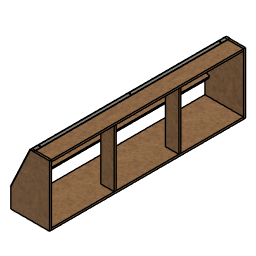
tricoro_panel (Autodesk Fusion 360 design; units mm, degrees)
Autodesk Fusion 360 part; units mm, degrees
note: some values were not read from the file. Set by a fixed rule: which sketch regions a step uses.
sketch "Sketch1" plane through (0, 0, 0) normal (0, 1, 0) x (1, 0, 0)
  line L0 (0, 0) -> (18, 0)
  line L1 (0, 0) -> (-101.4284, 217.5139)
  line L2 (0, 0) -> (240, 0) construction
  line L3 (-1.2741, -2) -> (-103.241, 216.6686)
  line L4 (-1.2741, -2) -> (18, -2)
  line L5 (18, -2) -> (18, 0)
  line L6 (-103.241, 216.6686) -> (-101.4284, 217.5139)
  dimension "d1" = 18
  dimension "d2" = 115
  dimension "d3" = 240
  dimension "d4" = -2
  constraint coincident L0.start L1.start
  constraint horizontal L0
  constraint horizontal L2
  constraint perpendicular L2 L5
  constraint perpendicular L1 L6
  measures "d1" distance of L0.start L0.end
  measures "d2" angle of L1 L2
  measures "d3" distance of L0.start L1.end
extrude "Extrude1" add sketch "Sketch1" along normal blind 1020 makes body 1
sketch "Sketch2" plane through (0, 0, 0) normal (0, -1, 0) x (1, 0, 0)
  line L0 (18, 2) -> (-1.2741, 2)
  line L1 (-1.2741, 2) -> (-103.241, -216.6686)
  line L2 (-103.241, -216.6686) -> (-101.4284, -217.5139)
  line L3 (-101.4284, -217.5139) -> (0, 0)
  line L4 (0, 0) -> (18, 0)
  line L5 (18, 0) -> (18, 2)
  line L6 (0, 0) -> (100, 0)
  line L7 (100, 0) -> (100, -220)
  line L8 (100, -220) -> (0, -220)
  line L9 (0, -220) -> (0, 0)
  line L10 (0, 0) -> (-101.4284, 0)
  line L11 (-101.4284, 0) -> (-101.4284, -217.5139)
  line L12 (-101.4284, -217.5139) -> (0, -217.5139)
  line L13 (0, -217.5139) -> (0, 0)
  line L14 (-101.4284, -217.5139) -> (100, -217.5139)
  line L15 (100, -217.5139) -> (100, -317.5139)
  line L16 (100, -317.5139) -> (-101.4284, -317.5139)
  line L17 (-101.4284, -317.5139) -> (-101.4284, -217.5139)
  dimension "d7" = 100
  dimension "d8" = 100
  constraint horizontal L6
  constraint vertical L7
  constraint horizontal L8
  constraint vertical L9
  constraint coincident L3.end L4.start
  constraint horizontal L10
  constraint vertical L11
  constraint horizontal L12
  constraint vertical L13
  constraint coincident L2.end L3.start
  constraint horizontal L14
  constraint vertical L15
  constraint horizontal L16
  constraint vertical L17
  measures "d7" distance of L3.end L6.end
  measures "d8" distance of L2.end L16.end
extrude "Extrude2" add sketch "Sketch2" against normal blind 10 separate body contours L4 L6 L7 L9 L13 L14 | L3 L9 L12 L13 L14 | L8 L9 L12 L14 L15 L16 L17 | L7 L8 L9 L14 L15 makes body 2
copy_body "CopyPasteBodies1" bodies 2 makes body 3
move_body "Move1" bodies 3 to x (1, 0, 0) y (0, 1, 0) z (0, 0, 1) at (0, 1010, 0)
sketch "Sketch3" plane through (0, 1010, 0) normal (0, -1, 0) x (1, 0, 0)
  line L0 (-101.4284, -317.5139) -> (100, -317.5139)
  line L1 (100, -317.5139) -> (100, 0)
  line L2 (100, 0) -> (0, 0)
  line L3 (0, 0) -> (-101.4284, -217.5139)
  line L4 (-101.4284, -217.5139) -> (-101.4284, -317.5139)
  line L5 (-101.4284, -217.5139) -> (-83.3022, -225.9662)
  line L6 (-83.3022, -225.9662) -> (-76.963, -212.3716)
  line L7 (-76.963, -212.3716) -> (-95.0891, -203.9193)
  line L8 (-95.0891, -203.9193) -> (-101.4284, -217.5139)
  dimension "d11" = 20
  dimension "d12" = 15
  constraint coincident L3.end L4.start
  constraint perpendicular L3 L5
  constraint perpendicular L5 L6
  constraint coincident L3 L7.end
  constraint perpendicular L3 L7
  measures "d11" distance of L3.end L5.end
  measures "d12" distance of L5.end L6.end
extrude "Extrude3" add sketch "Sketch3" along normal blind 1000 separate body contours L3 L5 L6 L7 L8 makes body 4
sketch "Sketch4" plane through (0, 1010, 0) normal (0, -1, 0) x (1, 0, 0)
  line L0 (-101.4284, -317.5139) -> (100, -317.5139)
  line L1 (100, -317.5139) -> (100, 0)
  line L2 (100, 0) -> (0, 0)
  line L3 (0, 0) -> (-101.4284, -217.5139)
  line L4 (-101.4284, -217.5139) -> (-101.4284, -317.5139)
  line L5 (100, 0) -> (0, 0)
  line L6 (0, 0) -> (0, -10)
  line L7 (0, -10) -> (100, -10)
  line L8 (100, -10) -> (100, 0)
  constraint horizontal L5
  constraint vertical L6
  constraint horizontal L7
  constraint vertical L8
  constraint coincident L1.end L2.start
extrude "Extrude4" add sketch "Sketch4" along normal blind 1000 separate body contours L1 L2 L5 L6 L7 L8 makes body 5
sketch "Sketch5" plane through (0, 1010, 0) normal (0, -1, 0) x (1, 0, 0)
  line L0 (-101.4284, -317.5139) -> (100, -317.5139)
  line L1 (100, -317.5139) -> (100, 0)
  line L2 (100, 0) -> (0, 0)
  line L3 (0, 0) -> (-101.4284, -217.5139)
  line L4 (-101.4284, -217.5139) -> (-101.4284, -317.5139)
  line L5 (100, -317.5139) -> (-101.4284, -317.5139)
  line L6 (-101.4284, -317.5139) -> (-101.4284, -307.5139)
  line L7 (-101.4284, -307.5139) -> (100, -307.5139)
  line L8 (100, -307.5139) -> (100, -317.5139)
  dimension "d17" = 10
  constraint horizontal L5
  constraint vertical L6
  constraint horizontal L7
  constraint vertical L8
  constraint coincident L0.end L1.start
  measures "d17" distance of L0.end L7.end
extrude "Extrude5" add sketch "Sketch5" along normal blind 1000 separate body contours L0 L1 L4 L5 L6 L7 L8 makes body 6
sketch "Sketch6" plane through (100, 0, 0) normal (1, 0, 0) x (0, 1, 0)
  line L0 (0, 0) -> (0, -317.5139)
  line L1 (0, -317.5139) -> (10, -317.5139)
  line L2 (10, -317.5139) -> (10, 0)
  line L3 (10, 0) -> (0, 0)
  line L4 (10, -10) -> (0, -10)
  line L5 (0, -10) -> (0, -307.5)
  line L6 (0, -307.5) -> (10, -307.5)
  line L7 (10, -307.5) -> (10, -10)
  line L8 (336.6667, -307.5) -> (346.6667, -307.5)
  line L9 (346.6667, -307.5) -> (346.6667, -10)
  line L10 (336.6667, -10) -> (336.6667, -307.5)
  line L11 (346.6667, -10) -> (336.6667, -10)
  line L12 (346.6667, 0) -> (336.6667, 0)
  line L13 (673.3333, -307.5) -> (683.3333, -307.5)
  line L14 (683.3333, -307.5) -> (683.3333, -10)
  line L15 (673.3333, -10) -> (673.3333, -307.5)
  line L16 (683.3333, -10) -> (673.3333, -10)
  line L17 (683.3333, 0) -> (673.3333, 0)
  line L18 (1010, -307.5) -> (1020, -307.5)
  line L19 (1020, -307.5) -> (1020, -10)
  line L20 (1010, -10) -> (1010, -307.5)
  line L21 (1020, -10) -> (1010, -10)
  line L22 (1020, 0) -> (1010, 0)
  point P0 (336.6667, 0)
  point P1 (673.3333, 0)
  point P2 (1010, 0)
  dimension "d22" = 1010
  dimension "d23" = 0
  constraint horizontal L4
  constraint vertical L5
  constraint horizontal L6
  constraint vertical L7
  constraint coincident L0 L5.end
  constraint coincident L2 L4.start
extrude "Extrude6" add sketch "Sketch6" against normal blind 70 separate body contours L8 L9 L10 L11 | L13 L14 L15 L16 makes body 7 at (76.6667, 336.6667, -109.1667) makes body 8 at (76.6667, 673.3333, -109.1667)
sketch "Sketch7" plane through (0, 0, 2) normal (0, 0, 1) x (-1, 0, 0)
  line L0 (1.2741, 0) -> (-18, 0)
  line L1 (-18, 0) -> (-18, -1020)
  line L2 (-18, -1020) -> (1.2741, -1020)
  line L3 (1.2741, -1020) -> (1.2741, 0)
  line L4 (-18, 0) -> (-8, 0)
  line L5 (-8, 0) -> (-8, -40)
  line L6 (-8, -40) -> (-18, -40)
  line L7 (-18, -40) -> (-18, 0)
  circle A0 centre (-8, -40) radius 3
  circle A1 centre (-8, -510) radius 3
  circle A2 centre (-8, -980) radius 3
  point P0 (-8, -510)
  point P1 (-8, -980)
  dimension "d26" = 10
  dimension "d27" = 40
  dimension "d30" = 0
  dimension "d31" = -940
  constraint horizontal L4
  constraint vertical L5
  constraint horizontal L6
  constraint vertical L7
  constraint coincident L0.end L1.start
  constraint coincident L5.end L6.start
  measures "d26" distance of L0.end L4.end
  measures "d27" distance of L0.end L6.end
extrude "Extrude7" cut sketch "Sketch7" against normal blind 20 contours L5 L6 A0 | L5 L6 A0 | A1 | A2 bodies 1 5
fillet "Fillet1" radius 5 1 edges at (-1.2741, 510, 2) on bodies 1
sketch "Sketch8" plane through (-1.8126, 0, 0.8452) normal (-0.906308, 0, 0.422618) x (0, -1, 0)
  line L0 (0, -1.9112) -> (-1020, -1.9112)
  line L1 (-1020, -1.9112) -> (-1020, -240)
  line L2 (-1020, -240) -> (0, -240)
  line L3 (0, -240) -> (0, -1.9112)
  line L4 (0, -240) -> (-40, -240)
  line L5 (-40, -240) -> (-40, -230)
  line L6 (-40, -230) -> (0, -230)
  line L7 (0, -230) -> (0, -240)
  circle A0 centre (-40, -230) radius 3
  circle A1 centre (-353.3333, -230) radius 3
  circle A2 centre (-666.6667, -230) radius 3
  circle A3 centre (-980, -230) radius 3
  dimension "d36" = 40
  dimension "d37" = 10
  dimension "d38" = 6
  dimension "d41" = -940
  dimension "d42" = 0
  constraint horizontal L4
  constraint vertical L5
  constraint horizontal L6
  constraint vertical L7
  constraint coincident L2.end L3.start
  constraint coincident L5.end L6.start
  measures "d36" distance of L2.end L4.end
  measures "d37" distance of L2.end L6.end
  measures "d38" diameter of A0
extrude "Extrude8" cut sketch "Sketch8" against normal blind 70 contours L5 L6 A0 | L5 L6 A0 | A1 | A2 | A3 bodies 1 4
